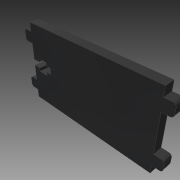
# Autodesk Inventor part: spool_brace
Saved by Autodesk Inventor 2014 (Build 180170000, 170)
## iProperties
Created: 2014-04-05
Part Number: spool_brace
Material: Plywood, Finish
Document SubType Name: Modeling
Designer: buben
Density: 0.552 g/cm^3
Appearance: Anodized - Dark Gray
Author: buben
Autodesk Inventor part; units mm, degrees
ref_plane "YZ Plane" through (0, 0, 0) normal (1, 0, 0) x (0, 1, 0)
ref_plane "XZ Plane" through (0, 0, 0) normal (0, 1, 0) x (-1, 0, 0)
ref_plane "XY Plane" through (0, 0, 0) normal (0, 0, 1) x (1, 0, 0)
sketch "Sketch1" plane through (0, 0, 0) normal (0, 1, 0) x (-1, 0, 0)
  line L0 (0, 0) -> (-95, 0)
  line L1 (-95, 0) -> (-95, -55)
  line L2 (-95, -55) -> (0, -55)
  line L3 (0, -55) -> (0, 0)
  dimension "d0" = 55
  dimension "d1" = 95
  constraints: 8 end point, 2 parallel, 1 horizontal, 1 perpendicular
  measures "d0" distance of L2.end L0.start
  measures "d1" distance of L0.start L0.end
extrude "Extrusion1" add sketch "Sketch1" along normal blind 6.5
sketch "Sketch3" plane through (0, 6.5, 0) normal (0, 1, 0) x (1, 0, 0)
  line L0 (0, 0) -> (95, 0) projected
  line L1 (95, 55) -> (0, 55) projected
  line L2 (0, 55) -> (0, 0) projected
  line L3 (0, 49) -> (-4.5, 49)
  line L4 (-6.5, 47) -> (-6.5, 43)
  line L5 (-4.5, 41) -> (0, 41)
  line L6 (0, 41) -> (0, 49)
  line L7 (47.5, 55) -> (47.5, 0) construction
  line L8 (0, 14) -> (-4.5, 14)
  line L9 (-6.5, 12) -> (-6.5, 8)
  line L10 (-4.5, 6) -> (0, 6)
  line L11 (0, 6) -> (0, 14)
  arc A0 (-4.5, 49) -> (-6.5, 47) centre (-4.5, 47) ccw
  arc A1 (-6.5, 43) -> (-4.5, 41) centre (-4.5, 43) ccw
  arc A2 (-4.5, 14) -> (-6.5, 12) centre (-4.5, 12) ccw
  arc A3 (-6.5, 8) -> (-4.5, 6) centre (-4.5, 8) ccw
  line L12 (95, 49) -> (99.5, 49)
  line L13 (101.5, 47) -> (101.5, 43)
  line L14 (99.5, 41) -> (95, 41)
  line L15 (95, 41) -> (95, 49)
  line L16 (95, 14) -> (99.5, 14)
  line L17 (101.5, 12) -> (101.5, 8)
  line L18 (99.5, 6) -> (95, 6)
  line L19 (95, 6) -> (95, 14)
  arc A4 (101.5, 47) -> (99.5, 49) centre (99.5, 47) ccw
  arc A5 (99.5, 41) -> (101.5, 43) centre (99.5, 43) ccw
  arc A6 (101.5, 12) -> (99.5, 14) centre (99.5, 12) ccw
  arc A7 (99.5, 6) -> (101.5, 8) centre (99.5, 8) ccw
  dimension "d13" = 2
  dimension "d14" = 8
  dimension "d15" = 8
  dimension "d16" = 6.5
  dimension "d17" = 6
  dimension "d18" = 6
  constraints: 34 end point, 16 point on circle, 16 symmetric about line, 8 centre point, 8 tangent, 4 parallel, 3 equal radius, 2 horizontal, 2 midpoint, 2 perpendicular, 2 point on line, 1 collinear, 4 other
  measures "d13" radius of A0
  measures "d14" distance between parallel lines of L5 L3
  measures "d15" distance between parallel lines of L10 L8
  measures "d16" distance between parallel lines of L6 L4
  measures "d17" distance between parallel lines of L0 L10
  measures "d18" distance between parallel lines of L1 L3
extrude "Extrusion3" add sketch "Sketch3" against normal blind 6.5
sketch "Sketch4" plane through (0, 0, 0) normal (0, -1, 0) x (1, 0, 0)
  line L0 (0, -41) -> (0, -14) projected
  line L1 (16.3, -25.25) -> (16.3, -29.75)
  line L2 (0, -29.75) -> (0, -25.25)
  line L3 (5, -22.75) -> (12.3, -22.75)
  line L4 (12.3, -32.25) -> (5, -32.25)
  line L5 (0, -25.25) -> (5, -25.25)
  line L6 (12.3, -25.25) -> (16.3, -25.25)
  line L7 (16.3, -29.75) -> (12.3, -29.75)
  line L8 (5, -29.75) -> (0, -29.75)
  line L9 (5, -32.25) -> (5, -29.75)
  line L10 (5, -25.25) -> (5, -22.75)
  line L11 (12.3, -22.75) -> (12.3, -25.25)
  line L12 (12.3, -29.75) -> (12.3, -32.25)
  point P0 (0, -27.5)
  dimension "d21" = 4.5
  dimension "d22" = 5
  dimension "d23" = 4
  dimension "d24" = 7.3
  dimension "d25" = 2.5
  constraints: 24 end point, 10 parallel, 5 collinear, 4 perpendicular, 3 horizontal, 2 midpoint
  measures "d21" distance of L1.start L1.end
  measures "d22" distance of L8.start L2.start
  measures "d23" distance of L1.end L7.end
  measures "d24" distance of L4.start L4.end
  measures "d25" distance of L7.end L4.start
extrude "Extrusion4" cut sketch "Sketch4" against normal through all
equation "\"d18\" = d17"
body "Solid1"
